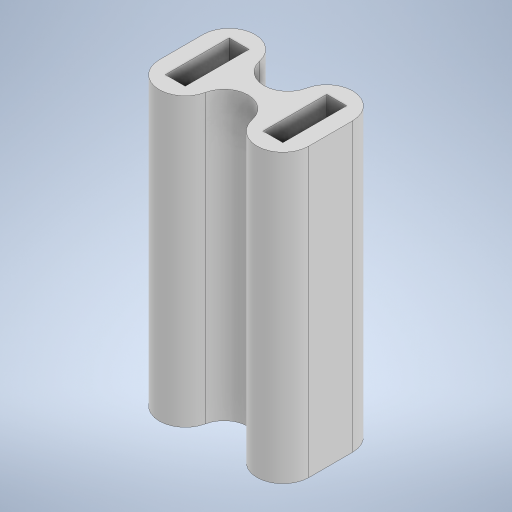
# Autodesk Inventor part: pilar soporte
Saved by Autodesk Inventor 2024 (Build 280153000, 153)
## iProperties
Created: 2024-04-30
Part Number: pilar soporte
Material: Generic
Document SubType Name: Modeling
Designer: JF Balaguer
Density: 1 g/cm^3
Appearance: Default
Author: JF Balaguer
Autodesk Inventor part; units mm, degrees
ref_plane "YZ Plane" through (0, 0, 0) normal (1, 0, 0) x (0, 1, 0)
ref_plane "XZ Plane" through (0, 0, 0) normal (0, 1, 0) x (-1, 0, 0)
ref_plane "XY Plane" through (0, 0, 0) normal (0, 0, 1) x (1, 0, 0)
sketch "Sketch1" plane through (0, 0, 0) normal (0, 1, 0) x (-1, 0, 0)
  line L0 (14.75, -8) -> (9.75, -8)
  line L1 (9.75, -8) -> (9.75, 8)
  line L2 (9.75, 8) -> (14.75, 8)
  line L3 (14.75, 8) -> (14.75, -8)
  line L4 (-14.75, -8) -> (-9.75, -8)
  line L5 (-9.75, -8) -> (-9.75, 8)
  line L6 (-9.75, 8) -> (-14.75, 8)
  line L7 (-14.75, 8) -> (-14.75, -8)
  line L8 (0, -17.6647) -> (0, 17.6647) projected
  line L9 (27.0734, 0) -> (-27.0734, 0) projected
  line L10 (18.75, -12) -> (-18.75, -12)
  line L11 (-18.75, -12) -> (-18.75, 12)
  line L12 (-18.75, 12) -> (18.75, 12)
  line L13 (18.75, 12) -> (18.75, -12)
  arc A0 (5.8816, -6.8013) -> (18.75, -5.5) centre (12.25, -5.5) ccw
  arc A1 (-18.75, -5.5) -> (-5.8816, -6.8013) centre (-12.25, -5.5) ccw
  arc A2 (5.8816, -6.8013) -> (-5.8816, -6.8013) centre (0, -8.0031) ccw
  arc A3 (18.75, 5.5) -> (5.8816, 6.8013) centre (12.25, 5.5) ccw
  arc A4 (-5.8816, 6.8013) -> (-18.75, 5.5) centre (-12.25, 5.5) ccw
  arc A5 (-5.8816, 6.8013) -> (5.8816, 6.8013) centre (0, 8.0031) ccw
  point P0 (0, 0)
  point P1 (0, -2)
  point P2 (-18.75, 5.5)
  dimension "d0" = 5
  dimension "d1" = 16
  dimension "d2" = 16
  dimension "d3" = 19.5
  dimension "d4" = 37.5
  dimension "d5" = 24
  dimension "d6" = 6.5
  dimension "d7" = 4
  dimension "d8" = 2
  constraints: 24 end point, 13 point on circle, 8 symmetric about line, 6 centre point, 6 parallel, 4 point on line, 3 horizontal, 3 perpendicular, 3 tangent, 10 other
  measures "d0" distance between parallel lines of L1 L3
  measures "d1" distance between parallel lines of L2 L0
  measures "d2" distance between parallel lines of L6 L4
  measures "d3" distance between parallel lines of L5 L1
  measures "d4" distance between parallel lines of L11 L13
  measures "d5" distance of L10.end L11.end
  measures "d6" distance from line of L13 A0.centre
  measures "d7" distance between parallel lines of L13 L3
  measures "d8" distance from line of L9 point (0, -2)
extrude "Extrusion1" add sketch "Sketch1" against normal blind 72 contours L3 L9 L13 A0 A2 L8 L1 L0 | L3 L2 L1 L9 L8 A5 A3 L13 | L9 L5 L6 L7 L11 A4 A5 L8 | L8 A2 A1 L11 L9 L7 L4 L5
sketch "Sketch2" plane through (0, -72, 0) normal (0, -1, 0) x (1, 0, 0)
  arc A0 (-5.8816, 6.8013) -> (-18.75, 5.5) centre (-12.25, 5.5) ccw projected
  line L0 (-18.75, 5.5) -> (-18.75, -5.5) projected
  arc A1 (-18.75, -5.5) -> (-5.8816, -6.8013) centre (-12.25, -5.5) ccw projected
  arc A2 (5.8816, -6.8013) -> (-5.8816, -6.8013) centre (0, -8.0031) ccw projected
  arc A3 (5.8816, -6.8013) -> (18.75, -5.5) centre (12.25, -5.5) ccw projected
  line L1 (18.75, -5.5) -> (18.75, 5.5) projected
  arc A4 (18.75, 5.5) -> (5.8816, 6.8013) centre (12.25, 5.5) ccw projected
  arc A5 (-5.8816, 6.8013) -> (5.8816, 6.8013) centre (0, 8.0031) ccw projected
  line L2 (-14.75, -8) -> (-14.75, 8) projected
  line L3 (-14.75, 8) -> (-9.75, 8) projected
  line L4 (-9.75, 8) -> (-9.75, -8) projected
  line L5 (-9.75, -8) -> (-14.75, -8) projected
  line L6 (9.75, -8) -> (9.75, 8) projected
  line L7 (9.75, 8) -> (14.75, 8) projected
  line L8 (14.75, 8) -> (14.75, -8) projected
  line L9 (14.75, -8) -> (9.75, -8) projected
  line L10 (15.9006, 9.0344) -> (8.0535, 9.0344)
  line L11 (8.0535, 9.0344) -> (8.0535, -9.2409)
  line L12 (8.0535, -9.2409) -> (15.9006, -9.2409)
  line L13 (15.9006, -9.2409) -> (15.9006, 9.0344)
  line L14 (-8.673, 9.0344) -> (-16.1071, 9.0344)
  line L15 (-16.1071, 9.0344) -> (-16.1071, -9.2409)
  line L16 (-16.1071, -9.2409) -> (-8.673, -9.2409)
  line L17 (-8.673, -9.2409) -> (-8.673, 9.0344)
  point P0 (0, 0)
  constraints: 16 end point, 4 parallel, 2 horizontal, 2 perpendicular, 2 point on line
extrude "Extrusion2" add sketch "Sketch2" against normal blind 56 contours L2 L3 L4 L5 | L6 L7 L8 L9 | L13 L12 L11 L10 | L17 L16 L15 L14
body "Solid1"
